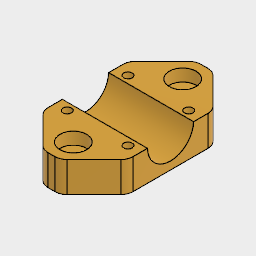
Y_Carriage_Clamp_1.0_F01 (Autodesk Fusion 360 design; units mm, degrees)
Autodesk Fusion 360 part; units mm, degrees
note: some values were not read from the file. Set by a fixed rule: which sketch regions a step uses.
sketch "スケッチ1" plane through (0, 0, 0) normal (0, 0, 1) x (1, 0, 0)
  line L0 (-3.5, 31.5) -> (3.5, 31.5)
  line L1 (3.5, 31.5) -> (17.5, 17.5)
  line L2 (17.5, 17.5) -> (17.5, -17.5)
  line L3 (17.5, -17.5) -> (3.5, -31.5)
  line L4 (3.5, -31.5) -> (-3.5, -31.5)
  line L5 (-3.5, -31.5) -> (-17.5, -17.5)
  line L6 (-17.5, -17.5) -> (-17.5, 17.5)
  line L7 (-17.5, 17.5) -> (-3.5, 31.5)
  circle A0 centre (-12.5, 12.5) radius 3
  circle A1 centre (-12.5, -12.5) radius 3
  circle A2 centre (12.5, -12.5) radius 3
  circle A3 centre (12.5, 12.5) radius 3
  dimension "d1" = 35
  dimension "d2" = 63
  dimension "d3" = 31.5
  dimension "d4" = 17.5
  dimension "d5" = 14
  dimension "d6" = 14
  dimension "d7" = 14
  dimension "d8" = 14
  dimension "d9" = 14
  dimension "d10" = 14
  dimension "d11" = 14
  dimension "d12" = 14
  dimension "d13" = 6
  dimension "d14" = 12.5
  dimension "d15" = 12.5
  dimension "d17" = 360
  measures "d1" distance of L2 L6
  measures "d2" distance of L0 L4
  measures "d3" distance of origin L0
  measures "d4" distance of origin L6
  measures "d5" distance of L0.start L6.end
  measures "d6" distance of L0.start L6.end
  measures "d7" distance of L0.end L1.end
  measures "d8" distance of L0.end L1.end
  measures "d9" distance of L2.end L3.end
  measures "d10" distance of L2.end L3.end
  measures "d11" distance of L4.end L5.end
  measures "d12" distance of L4.end L5.end
  measures "d13" diameter of A0
  measures "d14" distance of origin A0.centre
  measures "d15" distance of origin A0.centre
extrude "押し出し1" add sketch "スケッチ1" along normal blind 12.5 contours L0 L1 L2 L3 L4 L5 L6 L7 | A0 | A1 | A2 | A3
extrude "押し出し2" cut sketch "スケッチ1" along normal blind 3 contours A0 | A1 | A2 | A3
sketch "スケッチ2" plane through (17.5, 0, 0) normal (1, 0, 0) x (0, 1, 0)
  line L0 (-17.5, 0) -> (17.5, 0)
  line L1 (17.5, 0) -> (17.5, 12.5)
  line L2 (17.5, 12.5) -> (-17.5, 12.5)
  line L3 (-17.5, 12.5) -> (-17.5, 0)
  circle A0 centre (0, 12.75) radius 9.5
  line L4 (17.5, 0) -> (-17.5, 0)
  dimension "d22" = 19
  dimension "d23" = 12.75
  measures "d22" diameter of A0
  measures "d23" distance of A0.centre L4
extrude "押し出し3" cut sketch "スケッチ2" against normal up to surface (35 mm away) contours L2 A0 picked at (1.5592, 9.8271)
sketch "スケッチ3" plane through (0, 0, 12.5) normal (0, 0, 1) x (-1, 0, 0)
  line L0 (17.5, -9.4967) -> (-17.5, -9.4967)
  line L1 (-17.5, -9.4967) -> (-17.5, -17.5)
  line L2 (-17.5, -17.5) -> (-3.5, -31.5)
  line L3 (-3.5, -31.5) -> (3.5, -31.5)
  line L4 (3.5, -31.5) -> (17.5, -17.5)
  line L5 (17.5, -17.5) -> (17.5, -9.4967)
  circle A0 centre (12.5, -12.5) radius 1.75
  circle A1 centre (12.5, 12.5) radius 1.75
  circle A2 centre (-12.5, 12.5) radius 1.75
  circle A3 centre (-12.5, -12.5) radius 1.75
  line L6 (-3.5, 31.5) -> (3.5, 31.5)
  line L7 (0, 31.5) -> (0, -31.5) construction
  circle A4 centre (0, 22.5) radius 5.5
  circle A5 centre (0, -22.5) radius 5.5
  point P0 (12.5, -12.5)
  dimension "d26" = 3.5
  dimension "d28" = 360
  dimension "d32" = 11
  dimension "d33" = 11
  dimension "d34" = 9
  dimension "d35" = 9
  measures "d26" diameter of A0
  measures "d32" diameter of A4
  measures "d33" diameter of A5
  measures "d34" distance of L6 A4.centre
  measures "d35" distance of L3 A5.centre
extrude "押し出し4" cut sketch "スケッチ3" against normal blind 9.1 contours A0 | A1 | A2 | A3
extrude "押し出し5" cut sketch "スケッチ3" against normal blind 5 contours A4 | A5
fillet "フィレット1" radius 5 8 edges at (-17.5, 17.5, 6.25) (-3.5, 31.5, 6.25) (3.5, 31.5, 6.25) (17.5, 17.5, 6.25) (-17.5, -17.5, 6.25) (-3.5, -31.5, 6.25) (3.5, -31.5, 6.25) (17.5, -17.5, 6.25)
equation "d3 = d2 / 2"
equation "d4 = d1 / 2"
equation "d7 = d5"
equation "d8 = d6"
equation "d9 = d5"
equation "d10 = d7"
equation "d11 = d10"
equation "d12 = d9"
